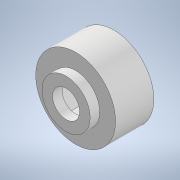
# Autodesk Inventor part: gear1
Saved by Autodesk Inventor 2022 (Build 260153000, 153)
## iProperties
Created: 2022-05-06
Part Number: gear1
Material: Generic
Document SubType Name: Modeling
Designer: erasm
Density: 1 g/cm^3
Appearance: Default
Author: erasm
Autodesk Inventor part; units mm, degrees
ref_plane "YZ Plane" through (0, 0, 0) normal (1, 0, 0) x (0, 1, 0)
ref_plane "XZ Plane" through (0, 0, 0) normal (0, 1, 0) x (-1, 0, 0)
ref_plane "XY Plane" through (0, 0, 0) normal (0, 0, 1) x (1, 0, 0)
sketch "Sketch1" plane through (0, 0, 0) normal (0, 0, 1) x (1, 0, 0)
  line L0 (-14.3448, 13.9006) -> (-7.8021, 17.4592)
  line L1 (-14.3448, 13.9006) -> (-14.5342, 6.4551)
  line L2 (-14.5342, 6.4551) -> (-8.1811, 2.5683)
  line L3 (-8.1811, 2.5683) -> (-1.6384, 6.127)
  line L4 (-1.4489, 13.5724) -> (-1.6384, 6.127)
  line L5 (-7.8021, 17.4592) -> (-1.4489, 13.5724)
  circle A0 centre (-8, 10) radius 4
  circle A1 centre (-8, 10) radius 7.5414
  line L6 (-4.1827, 16.5039) -> (-0.4588, 9.9461)
  line L7 (-0.4588, 9.9461) -> (-4.2761, 3.4422)
  line L8 (-4.2761, 3.4422) -> (-11.8173, 3.4961)
  line L9 (-11.8173, 3.4961) -> (-15.5412, 10.0539)
  line L10 (-15.5412, 10.0539) -> (-11.7239, 16.5578)
  line L11 (-11.7239, 16.5578) -> (-4.1827, 16.5039)
  circle A2 centre (-8, 10) radius 4.25
  circle A3 centre (-8, 10) radius 12.5
  point P0 (0, 0)
extrude "Extrusion1" add sketch "Sketch1" along normal blind 12 contours L1 L10 A1 L0 | L0 L10 L1 | L11 A1 L5 L0 | L0 L5 L11 | L9 L2 L1 | L1 L2 L9 A1 | A1 L6 L4 L5 | L8 L2 L3 A1 | L5 L4 L6 | L8 L3 L2 | L7 L3 L4 A1 | L7 L4 L3 | A3
sketch "Sketch2" plane through (-8, 10, 12) normal (0, 0, 1) x (1, 0, 0)
  circle A0 centre (0, 0) radius 4.25
  line L0 (7.5412, -0.0539) -> (3.7239, -6.5578) projected
  circle A1 centre (0, 0) radius 7.5414
  point P0 (8, -10)
  dimension "d4" = 8.5
  constraints: 1 centre point, 1 coincident, 3 other
  measures "d4" diameter of A0
extrude "Extrusion2" add sketch "Sketch2" along normal blind 3
body "Solid1"
